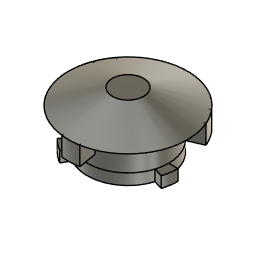
Safety Cap (Autodesk Fusion 360 design; units mm, degrees)
Autodesk Fusion 360 part; units mm, degrees
sketch "Sketch1" plane through (0, 0, 0) normal (0, 0, 1) x (1, 0, 0)
  circle A0 centre (0, 0) radius 16
  line L0 (-13.0228, 10.9274) -> (0, 0)
  line L1 (8.5, 14.7224) -> (0, 0)
  line L2 (-2.952, -16.7417) -> (0, 0)
  line L3 (0, 0) -> (-3.5992, 15.5899)
  line L4 (13.0228, 10.9274) -> (0, 0)
  line L5 (0, 0) -> (-11.7017, -10.912)
  line L6 (8.5, -14.7224) -> (0, 0)
  line L7 (17, 0) -> (0, 0)
  line L8 (-8.5, 14.7224) -> (0, 0)
  line L9 (0, 0) -> (15.3009, -4.6779)
  line L10 (15.9748, 5.8143) -> (0, 0)
  line L11 (-15.9748, 5.8143) -> (0, 0)
  line L12 (-17, 0) -> (0, 0)
  line L13 (2.952, -16.7417) -> (0, 0)
  line L14 (0, -16) -> (0, 0)
  circle A1 centre (0, 0) radius 10
  circle A2 centre (0, 0) radius 17
  line L15 (-8.5, -14.7224) -> (0, 0)
  circle A3 centre (0, 0) radius 13
  circle A4 centre (0, 0) radius 5.5
  dimension "d36" = 360
  dimension "d38" = 360
  dimension "d39" = 26
  dimension "d40" = 20
  dimension "d41" = 17
  dimension "d42" = 60
  dimension "d44" = 11
  dimension "d45" = 32
  constraint coincident L14.start A0
  constraint vertical L14
  constraint concentric A1 A2
  constraint coincident A0.centre L14
  constraint coincident L6.start A2
  constraint coincident A0.centre L6
  constraint concentric A2 A3
  constraint symmetric L15.start L6.start L14
  constraint coincident L13.start A2
  constraint coincident A0.centre L13
  constraint symmetric A0.centre L0.end L14
  constraint symmetric L2.start L13.start L14
  constraint coincident A0.centre L0.end
  constraint coincident L5.end A0
  measures "d39" diameter of A3
  measures "d40" angle of L6 L13
  measures "d41" angle of L5 L15
  measures "d42" angle of L6 L15
  measures "d44" diameter of A4
  measures "d45" diameter of A0
extrude "Extrude1" add sketch "Sketch1" along normal blind 3.5 contours A0 L7 L9 A3 | L6 L9 A1 A3 | L7 L9 A1 A3 | L7 L10 A1 A3 | L6 L13 A1 A3 | L6 L9 A1 A4 | L7 L9 A1 A4 | L4 L10 A1 A3 | L7 L10 A1 A4 | L13 L14 A1 A3 | L6 L13 A1 A4 | L1 L4 A1 A3 | L4 L10 A1 A4 | L2 L14 A1 A3 | L13 L14 A1 A4 | A0 L3 L8 A3 | L1 L3 A1 A3 | L1 L4 A1 A4 | A0 L5 L15 A3 | L2 A1 L15 A3 | L2 L14 A1 A4 | L0 L11 A1 A4 | L0 L8 A1 A4 | L1 L3 A1 A4 | L2 A1 L15 A4 | L3 L8 A1 A4 | L5 A1 L15 A4 | L5 L12 A1 A4 | L11 L12 A1 A4 | L3 L8 A1 A3 | L5 A1 L15 A3 | L0 L11 A1 A3 | L0 L8 A1 A3 | L5 L12 A1 A3 | L11 L12 A1 A3 makes body 1
sketch "Sketch2" plane through (0, 0, 3.5) normal (0, 0, 1) x (-1, 0, 0)
  circle A0 centre (0, -0.0008) radius 13
  circle A1 centre (0, -0.0008) radius 5.5
  line L0 (2.9244, -12.6668) -> (3.5992, -15.5899)
  arc A2 (3.5992, -15.5899) -> (8, -13.8564) centre (0, 0) ccw
  line L1 (8, -13.8564) -> (6.5, -11.2583)
  line L2 (-12.432, 3.8008) -> (-15.3009, 4.6779)
  arc A3 (-15.3009, 4.6779) -> (-16, 0) centre (0, 0) ccw
  line L3 (-16, 0) -> (-13, 0)
  arc A4 (-13, 0) -> (2.9244, -12.6668) centre (0, 0) ccw
  line L4 (9.5076, 8.866) -> (11.7017, 10.912)
  arc A5 (11.7017, 10.912) -> (8, 13.8564) centre (0, 0) ccw
  line L5 (8, 13.8564) -> (6.5, 11.2583)
  arc A6 (6.5, -11.2583) -> (9.5076, 8.866) centre (0, 0) ccw
  arc A7 (6.5, 11.2583) -> (-12.432, 3.8008) centre (0, 0) ccw
  circle A8 centre (0, 0) radius 5.5
  dimension "d17" = 11
  constraint concentric A0 A1
  measures "d17" diameter of A1
extrude "Extrude2" add sketch "Sketch2" along normal blind 2 contours A0 A4 A6 A7 bodies 1
sketch "Sketch3" plane through (0, 0, 5.5) normal (0, 0, 1) x (-1, 0, 0)
  circle A0 centre (0, -0.0008) radius 5.5
  circle A1 centre (0, -0.0008) radius 13
  circle A2 centre (0, -0.0008) radius 13
  constraint concentric A0 A2
extrude "Extrude3" add sketch "Sketch3" along normal blind 7.5 contours A0 | A1 A2 bodies 1
sketch "Sketch4" plane through (0, 0, 13) normal (0, 0, 1) x (-1, 0, 0)
  circle A0 centre (0, -0.0008) radius 13
  circle A1 centre (0, -0.0008) radius 19
  circle A2 centre (0, -0.0008) radius 5.5
  line L0 (0, -0.0008) -> (3.5992, -15.5907)
  circle A3 centre (0, -0.0008) radius 10
  line L1 (3.2993, 18.7105) -> (0, -0.0008)
  line L2 (13.8564, -8.0008) -> (0, -0.0008)
  line L3 (-19, -0.0008) -> (0, -0.0008)
  line L4 (19, -0.0008) -> (0, -0.0008)
  line L5 (0, -0.0008) -> (-15.3009, 4.6771)
  line L6 (-14.5548, -12.2138) -> (0, -0.0008)
  line L7 (-9.5, -16.4553) -> (0, -0.0008)
  line L8 (-17.8542, -6.4992) -> (0, -0.0008)
  circle A4 centre (0, -0.0008) radius 19
  line L9 (0, -0.0008) -> (11.7017, 10.9112)
  line L10 (9.5, 16.4537) -> (0, -0.0008)
  circle A5 centre (0, -0.0008) radius 13
  line L11 (17.8542, -6.4992) -> (0, -0.0008)
  line L12 (9.5, -16.4553) -> (0, -0.0008)
  line L13 (14.5548, -12.2138) -> (0, -0.0008)
  line L14 (-9.5, 16.4537) -> (0, -0.0008)
  circle A6 centre (0, -0.0008) radius 16
  line L15 (-3.2993, 18.7105) -> (0, -0.0008)
  line L16 (15.1741, -11.4353) -> (0, -0.0008)
  line L17 (2.3155, 18.8576) -> (0, -0.0008)
  line L18 (-17.4896, -7.4247) -> (0, -0.0008)
  point P0 (0, -0.0008)
  point P1 (0, -0.0008)
  point P2 (0, -0.0008)
  dimension "d25" = 38
  dimension "d47" = 360
  dimension "d49" = 360
  dimension "d50" = 26
  dimension "d51" = 20
  dimension "d52" = 17
  dimension "d53" = 60
  dimension "d54" = 11
  dimension "d55" = 32
  dimension "d57" = 23
  dimension "d59" = 360
  constraint concentric A0 A1
  constraint coincident L2.start A6
  constraint concentric A3 A4
  constraint coincident P2 L2
  constraint coincident L4.start A4
  constraint coincident P2 L4
  constraint concentric A4 A5
  constraint symmetric L4.start L12.start L2
  constraint coincident L11.start A4
  constraint coincident P2 L11
  constraint symmetric P2 P1 L2
  constraint symmetric L11.start L13.start L2
  constraint coincident P2 P1
  constraint coincident L0.end A6
  constraint equal A1 A4
  constraint coincident A1 L16.start
  constraint concentric A1 A6
  measures "d25" diameter of A1
  measures "d50" diameter of A5
  measures "d51" angle of L4 L11
  measures "d52" angle of L0 L12
  measures "d53" angle of L4 L12
  measures "d54" diameter of A2
  measures "d55" diameter of A6
  measures "d57" angle of L12 L16
ref_plane "WorkPlane1" through (0, 0.0008, 18) normal (0, 0, 1) x (-1, 0, 0)
sketch "Sketch5" plane through (0, 0, 18) normal (0, 0, 1) x (1, 0, 0)
  circle A0 centre (0, 0) radius 5
  constraint coincident A0.centre origin
loft "Loft1" add profiles "Sketch4", "Sketch5" section 1 section 2 bodies 1
ref_plane "WorkPlane2" through (0, 0, 12.125) normal (-1, 0, 0) x (0, 0, 1)
sketch "Sketch6" plane through (0, 0, 0) normal (-1, 0, 0) x (0, -1, 0)
  line L0 (-13, 0) -> (-4.8771, 3)
  line L1 (-4.8771, 3) -> (-4.8771, 0)
  line L2 (-4.8771, 0) -> (-13, 0)
  line L3 (-5.5008, 5.5) -> (5.4992, 5.5)
  dimension "d16" = 2.5
  constraint vertical L1
  constraint perpendicular L1 L2
  measures "d16" distance of L0.end L3
revolve "Revolve1" cut sketch "Sketch6" angle 360 about axis through (0, 0, 1.75) along (0, 0, 1) bodies 1
sketch "Sketch7" plane through (0, 0, 18) normal (0, 0, 1) x (-1, 0, 0)
  circle A0 centre (0, 0) radius 5
  circle A1 centre (0, 0) radius 0
  circle A2 centre (0, 0) radius 0.4
  dimension "Identifier" = 0
  dimension "d21" = 0.8
  constraint concentric A0 A1
  constraint concentric A0 A2
  measures "Identifier" diameter of A1
  measures "d21" diameter of A2
extrude "Extrude5" add sketch "Sketch4" against normal blind 6 separate body contours A0 L2 A5 L11 A6 | A0 L2 A5 A6 L16 | A1 A4 L11 A6 L16 | A0 A5 A6 L15 L17 | A1 A4 A6 L15 L17 | A0 L6 A5 A6 L18 | A1 L6 A4 A6 L18 makes body 2 at (15.6486, 6.6432, 11) makes body 3 at (-2.0718, -16.8725, 11) makes body 4 at (-15.9748, 5.8151, 9)
equation "Width = 11 mm"
equation "depth = 2 mm"
equation "d11 = 9 mm - depth + 0.5 mm"
equation "d16 = depth + 0.5 mm"
equation "d17 = Width"
equation "d21 = Identifier + 0.8 mm"
